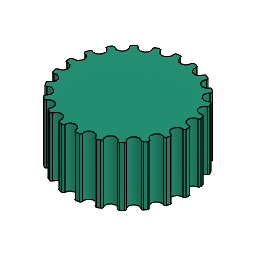
22T Pulley template v2 (Autodesk Fusion 360 design; units mm, degrees)
Autodesk Fusion 360 part; units mm, degrees
sketch "Sketch1" plane through (0, 0, 0) normal (0, 0, 1) x (1, 0, 0) in component "22T Pulley"
  circle A0 centre (0, 0) radius 10.125 construction
  circle A1 centre (0, 0) radius 8.925 construction
  line L0 (0, 0) -> (0, 8.925) construction
  circle A2 centre (0, 9.815) radius 0.89 construction
  circle A3 centre (1.14, 9.809) radius 0.25 construction
  line L1 (0, 0) -> (3.8847, 13.2301) construction
  line L2 (0, 0) -> (13.7887, 0) construction
  circle A4 centre (2.7652, 9.4174) radius 0.89 construction
  circle A5 centre (1.6697, 9.7328) radius 0.25 construction
  arc A6 (0, 8.925) -> (0.89, 9.8103) centre (0, 9.815) ccw
  arc A7 (1.9099, 9.6637) -> (2.5145, 8.5635) centre (2.7652, 9.4174) ccw
  arc A8 (1.9099, 9.6637) -> (1.712, 9.9792) centre (1.6697, 9.7328) ccw
  arc A9 (1.1756, 10.0564) -> (0.89, 9.8103) centre (1.14, 9.809) ccw
  line L3 (1.1756, 10.0564) -> (1.712, 9.9792)
  arc A10 (-2.5145, 8.5635) -> (-1.9099, 9.6637) centre (-2.7652, 9.4174) ccw
  arc A11 (-1.7052, 9.9803) -> (-1.9099, 9.6637) centre (-1.6697, 9.7328) ccw
  line L4 (-1.7052, 9.9803) -> (-1.1688, 10.0573)
  arc A12 (-0.89, 9.8103) -> (-1.1688, 10.0573) centre (-1.14, 9.809) ccw
  arc A13 (-0.89, 9.8103) -> (0, 8.925) centre (0, 9.815) ccw
  arc A14 (-4.8252, 7.5082) -> (-4.5551, 8.7341) centre (-5.3064, 8.2569) ccw
  arc A15 (-4.4479, 9.0956) -> (-4.5551, 8.7341) centre (-4.3441, 8.8682) ccw
  line L5 (-4.4479, 9.0956) -> (-3.955, 9.3206)
  arc A16 (-3.6178, 9.1622) -> (-3.955, 9.3206) centre (-3.8573, 9.0905) ccw
  arc A17 (-3.6178, 9.1622) -> (-2.5145, 8.5635) centre (-2.7652, 9.4174) ccw
  arc A18 (-6.7451, 5.8446) -> (-6.8313, 7.097) centre (-7.4177, 6.4275) ccw
  arc A19 (-6.8303, 7.474) -> (-6.8313, 7.097) centre (-6.6666, 7.2851) ccw
  line L6 (-6.8303, 7.474) -> (-6.4207, 7.8288)
  arc A20 (-6.0526, 7.7718) -> (-6.4207, 7.8288) centre (-6.2621, 7.6355) ccw
  arc A21 (-6.0526, 7.7718) -> (-4.8252, 7.5082) centre (-5.3064, 8.2569) ccw
  arc A22 (-8.1185, 3.7076) -> (-8.554, 4.8849) centre (-8.928, 4.0773) ccw
  arc A23 (-8.6593, 5.247) -> (-8.554, 4.8849) centre (-8.449, 5.1118) ccw
  line L7 (-8.6593, 5.247) -> (-8.3662, 5.7028)
  arc A24 (-7.9969, 5.7518) -> (-8.3662, 5.7028) centre (-8.1597, 5.562) ccw
  arc A25 (-7.9969, 5.7518) -> (-6.7451, 5.8446) centre (-7.4177, 6.4275) ccw
  arc A26 (-8.8342, 1.2702) -> (-9.5838, 2.2771) centre (-9.7151, 1.3968) ccw
  arc A27 (-9.7868, 2.5948) -> (-9.5838, 2.2771) centre (-9.5469, 2.5243) ccw
  line L8 (-9.7868, 2.5948) -> (-9.634, 3.1147)
  arc A28 (-9.2935, 3.2658) -> (-9.634, 3.1147) centre (-9.3961, 3.0378) ccw
  arc A29 (-9.2935, 3.2658) -> (-8.1185, 3.7076) centre (-8.928, 4.0773) ccw
  arc A30 (-8.8342, -1.2702) -> (-9.8371, -0.5152) centre (-9.7151, -1.3968) ccw
  arc A31 (-10.1214, -0.2675) -> (-9.8371, -0.5152) centre (-9.8714, -0.2676) ccw
  line L9 (-10.1214, -0.2675) -> (-10.1213, 0.2744)
  arc A32 (-9.8371, 0.5152) -> (-10.1213, 0.2744) centre (-9.8714, 0.2676) ccw
  arc A33 (-9.8371, 0.5152) -> (-8.8342, 1.2702) centre (-9.7151, 1.3968) ccw
  arc A34 (-8.1185, -3.7076) -> (-9.2935, -3.2658) centre (-8.928, -4.0773) ccw
  arc A35 (-9.636, -3.1082) -> (-9.2935, -3.2658) centre (-9.3961, -3.0378) ccw
  line L10 (-9.636, -3.1082) -> (-9.7886, -2.5883)
  arc A36 (-9.5838, -2.2771) -> (-9.7886, -2.5883) centre (-9.5469, -2.5243) ccw
  arc A37 (-9.5838, -2.2771) -> (-8.8342, -1.2702) centre (-9.7151, -1.3968) ccw
  arc A38 (-6.7451, -5.8446) -> (-7.9969, -5.7518) centre (-7.4177, -6.4275) ccw
  arc A39 (-8.37, -5.6971) -> (-7.9969, -5.7518) centre (-8.1597, -5.562) ccw
  line L11 (-8.37, -5.6971) -> (-8.6629, -5.2412)
  arc A40 (-8.554, -4.8849) -> (-8.6629, -5.2412) centre (-8.449, -5.1118) ccw
  arc A41 (-8.554, -4.8849) -> (-8.1185, -3.7076) centre (-8.928, -4.0773) ccw
  arc A42 (-4.8252, -7.5082) -> (-6.0526, -7.7718) centre (-5.3064, -8.2569) ccw
  arc A43 (-6.4259, -7.8244) -> (-6.0526, -7.7718) centre (-6.2621, -7.6355) ccw
  line L12 (-6.4259, -7.8244) -> (-6.8354, -7.4695)
  arc A44 (-6.8313, -7.097) -> (-6.8354, -7.4695) centre (-6.6666, -7.2851) ccw
  arc A45 (-6.8313, -7.097) -> (-6.7451, -5.8446) centre (-7.4177, -6.4275) ccw
  arc A46 (-2.5145, -8.5635) -> (-3.6178, -9.1622) centre (-2.7652, -9.4174) ccw
  arc A47 (-3.9612, -9.3179) -> (-3.6178, -9.1622) centre (-3.8573, -9.0905) ccw
  line L13 (-3.9612, -9.3179) -> (-4.4541, -9.0927)
  arc A48 (-4.5551, -8.7341) -> (-4.4541, -9.0927) centre (-4.3441, -8.8682) ccw
  arc A49 (-4.5551, -8.7341) -> (-4.8252, -7.5082) centre (-5.3064, -8.2569) ccw
  arc A50 (0, -8.925) -> (-0.89, -9.8103) centre (0, -9.815) ccw
  arc A51 (-1.1756, -10.0564) -> (-0.89, -9.8103) centre (-1.14, -9.809) ccw
  line L14 (-1.1756, -10.0564) -> (-1.712, -9.9792)
  arc A52 (-1.9099, -9.6637) -> (-1.712, -9.9792) centre (-1.6697, -9.7328) ccw
  arc A53 (-1.9099, -9.6637) -> (-2.5145, -8.5635) centre (-2.7652, -9.4174) ccw
  arc A54 (2.5145, -8.5635) -> (1.9099, -9.6637) centre (2.7652, -9.4174) ccw
  arc A55 (1.7052, -9.9803) -> (1.9099, -9.6637) centre (1.6697, -9.7328) ccw
  line L15 (1.7052, -9.9803) -> (1.1688, -10.0573)
  arc A56 (0.89, -9.8103) -> (1.1688, -10.0573) centre (1.14, -9.809) ccw
  arc A57 (0.89, -9.8103) -> (0, -8.925) centre (0, -9.815) ccw
  arc A58 (4.8252, -7.5082) -> (4.5551, -8.7341) centre (5.3064, -8.2569) ccw
  arc A59 (4.4479, -9.0956) -> (4.5551, -8.7341) centre (4.3441, -8.8682) ccw
  line L16 (4.4479, -9.0956) -> (3.955, -9.3206)
  arc A60 (3.6178, -9.1622) -> (3.955, -9.3206) centre (3.8573, -9.0905) ccw
  arc A61 (3.6178, -9.1622) -> (2.5145, -8.5635) centre (2.7652, -9.4174) ccw
  arc A62 (6.7451, -5.8446) -> (6.8313, -7.097) centre (7.4177, -6.4275) ccw
  arc A63 (6.8303, -7.474) -> (6.8313, -7.097) centre (6.6666, -7.2851) ccw
  line L17 (6.8303, -7.474) -> (6.4207, -7.8288)
  arc A64 (6.0526, -7.7718) -> (6.4207, -7.8288) centre (6.2621, -7.6355) ccw
  arc A65 (6.0526, -7.7718) -> (4.8252, -7.5082) centre (5.3064, -8.2569) ccw
  arc A66 (8.1185, -3.7076) -> (8.554, -4.8849) centre (8.928, -4.0773) ccw
  arc A67 (8.6593, -5.247) -> (8.554, -4.8849) centre (8.449, -5.1118) ccw
  line L18 (8.6593, -5.247) -> (8.3662, -5.7028)
  arc A68 (7.9969, -5.7518) -> (8.3662, -5.7028) centre (8.1597, -5.562) ccw
  arc A69 (7.9969, -5.7518) -> (6.7451, -5.8446) centre (7.4177, -6.4275) ccw
  arc A70 (8.8342, -1.2702) -> (9.5838, -2.2771) centre (9.7151, -1.3968) ccw
  arc A71 (9.7868, -2.5948) -> (9.5838, -2.2771) centre (9.5469, -2.5243) ccw
  line L19 (9.7868, -2.5948) -> (9.634, -3.1147)
  arc A72 (9.2935, -3.2658) -> (9.634, -3.1147) centre (9.3961, -3.0378) ccw
  arc A73 (9.2935, -3.2658) -> (8.1185, -3.7076) centre (8.928, -4.0773) ccw
  arc A74 (8.8342, 1.2702) -> (9.8371, 0.5152) centre (9.7151, 1.3968) ccw
  arc A75 (10.1214, 0.2675) -> (9.8371, 0.5152) centre (9.8714, 0.2676) ccw
  line L20 (10.1214, 0.2675) -> (10.1213, -0.2744)
  arc A76 (9.8371, -0.5152) -> (10.1213, -0.2744) centre (9.8714, -0.2676) ccw
  arc A77 (9.8371, -0.5152) -> (8.8342, -1.2702) centre (9.7151, -1.3968) ccw
  arc A78 (8.1185, 3.7076) -> (9.2935, 3.2658) centre (8.928, 4.0773) ccw
  arc A79 (9.636, 3.1082) -> (9.2935, 3.2658) centre (9.3961, 3.0378) ccw
  line L21 (9.636, 3.1082) -> (9.7886, 2.5883)
  arc A80 (9.5838, 2.2771) -> (9.7886, 2.5883) centre (9.5469, 2.5243) ccw
  arc A81 (9.5838, 2.2771) -> (8.8342, 1.2702) centre (9.7151, 1.3968) ccw
  arc A82 (6.7451, 5.8446) -> (7.9969, 5.7518) centre (7.4177, 6.4275) ccw
  arc A83 (8.37, 5.6971) -> (7.9969, 5.7518) centre (8.1597, 5.562) ccw
  line L22 (8.37, 5.6971) -> (8.6629, 5.2412)
  arc A84 (8.554, 4.8849) -> (8.6629, 5.2412) centre (8.449, 5.1118) ccw
  arc A85 (8.554, 4.8849) -> (8.1185, 3.7076) centre (8.928, 4.0773) ccw
  arc A86 (4.8252, 7.5082) -> (6.0526, 7.7718) centre (5.3064, 8.2569) ccw
  arc A87 (6.4259, 7.8244) -> (6.0526, 7.7718) centre (6.2621, 7.6355) ccw
  line L23 (6.4259, 7.8244) -> (6.8354, 7.4695)
  arc A88 (6.8313, 7.097) -> (6.8354, 7.4695) centre (6.6666, 7.2851) ccw
  arc A89 (6.8313, 7.097) -> (6.7451, 5.8446) centre (7.4177, 6.4275) ccw
  arc A90 (2.5145, 8.5635) -> (3.6178, 9.1622) centre (2.7652, 9.4174) ccw
  arc A91 (3.9612, 9.3179) -> (3.6178, 9.1622) centre (3.8573, 9.0905) ccw
  line L24 (3.9612, 9.3179) -> (4.4541, 9.0927)
  arc A92 (4.5551, 8.7341) -> (4.4541, 9.0927) centre (4.3441, 8.8682) ccw
  arc A93 (4.5551, 8.7341) -> (4.8252, 7.5082) centre (5.3064, 8.2569) ccw
  dimension "d1" = 20.25
  dimension "d2" = 17.85
  dimension "d3" = 1.78
  dimension "d4" = 0.5
  dimension "d5" = 73.636
  dimension "d6" = 1.78
  dimension "d7" = 0.5
  dimension "d8" = 2.7936
  dimension "d10" = 360
  constraint coincident A0.centre A1.centre
  constraint coincident A1 L0.end
  constraint vertical L0
  constraint coincident L0.end A2
  constraint tangent A2 A3
  constraint tangent A0 A3
  constraint horizontal L2
  constraint tangent A4 A5
  constraint tangent A0 A5
  constraint coincident A1 A7.end
  constraint coincident L1 A7.end
  constraint coincident A4.centre A7.centre
  constraint coincident A3.centre A9.centre
  constraint tangent A2 A6
  constraint tangent A4 A7
  constraint tangent A5 A8
  constraint tangent A3 L3
  constraint tangent A4 A8
  measures "d1" diameter of A0
  measures "d2" diameter of A1
  measures "d3" diameter of A2
  measures "d4" diameter of A3
  measures "d5" angle of L1 L2
  measures "d6" diameter of A4
  measures "d7" diameter of A5
  measures "d8" distance of A2.centre A4.centre
extrude "Extrude1" add sketch "Sketch1" along normal blind 10
component "22T Pulley" placed x (1, 0, 0) y (0, 1, 0) z (0, 0, 1) at (0, 0, 0)
equation "d2 = d1 - ( ( 2 * 1.2 ) * 1 mm )"
equation "d5 = 90 deg - 16.36363636363636 deg"
equation "d6 = d3"
equation "d7 = d4"
